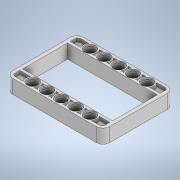
# Autodesk Inventor part: magazine-adapter
Saved by Autodesk Inventor 2021 (Build 250183000, 183)
## iProperties
Created: 2024-03-14
Part Number: magazine-adapter
Material: Generic
Document SubType Name: Modeling
Designer: 22hamfri
Density: 1 g/cm^3
Appearance: Default
Author: 22hamfri
Autodesk Inventor part; units mm, degrees
ref_plane "YZ Plane" through (0, 0, 0) normal (1, 0, 0) x (0, 1, 0)
ref_plane "XZ Plane" through (0, 0, 0) normal (0, 1, 0) x (-1, 0, 0)
ref_plane "XY Plane" through (0, 0, 0) normal (0, 0, 1) x (1, 0, 0)
sketch "Sketch1" plane through (0, 0, 0) normal (0, 1, 0) x (-1, 0, 0)
  line L0 (-25, 12.5) -> (25, 12.5)
  line L1 (25, 12.5) -> (25, -12.5)
  line L2 (25, -12.5) -> (-25, -12.5)
  line L3 (-25, -12.5) -> (-25, 12.5)
  line L4 (-25, 12.5) -> (25, -12.5) construction
  line L5 (25, 12.5) -> (-25, -12.5) construction
  line L6 (-27, 19.74) -> (27, 19.74)
  line L7 (27, 19.74) -> (27, -19.74)
  line L8 (27, -19.74) -> (-27, -19.74)
  line L9 (-27, -19.74) -> (-27, 19.74)
  line L10 (-27, 19.74) -> (27, -19.74) construction
  line L11 (27, 19.74) -> (-27, -19.74) construction
  circle A0 centre (0, -15.94) radius 2.575
  circle A1 centre (0, -15.94) radius 3.1
  circle A2 centre (0, -15.94) radius 3.8
  circle A3 centre (-7.97, -15.94) radius 2.575
  circle A4 centre (-7.97, -15.94) radius 3.1
  circle A5 centre (-7.97, -15.94) radius 3.8
  circle A6 centre (-15.94, -15.94) radius 2.575
  circle A7 centre (-15.94, -15.94) radius 3.1
  circle A8 centre (-15.94, -15.94) radius 3.8
  circle A9 centre (7.97, -15.94) radius 2.575
  circle A10 centre (7.97, -15.94) radius 3.1
  circle A11 centre (7.97, -15.94) radius 3.8
  circle A12 centre (0, -15.94) radius 2.575
  circle A13 centre (0, -15.94) radius 3.1
  circle A14 centre (0, -15.94) radius 3.8
  circle A15 centre (-7.97, -15.94) radius 2.575
  circle A16 centre (-7.97, -15.94) radius 3.1
  circle A17 centre (-7.97, -15.94) radius 3.8
  circle A18 centre (15.94, -15.94) radius 2.575
  circle A19 centre (15.94, -15.94) radius 3.1
  circle A20 centre (15.94, -15.94) radius 3.8
  circle A21 centre (7.97, -15.94) radius 2.575
  circle A22 centre (7.97, -15.94) radius 3.1
  circle A23 centre (7.97, -15.94) radius 3.8
  circle A24 centre (0, -15.94) radius 2.575
  circle A25 centre (0, -15.94) radius 3.1
  circle A26 centre (0, -15.94) radius 3.8
  line L12 (0, 0) -> (0, -19.74)
  line L13 (19.2075, -14) -> (25, -14)
  line L14 (25, -14) -> (25, -17.3718)
  line L15 (12.6725, -14) -> (11.2375, -14)
  line L16 (12.9151, -18.24) -> (10.9949, -18.24)
  line L17 (4.7025, -14) -> (3.2675, -14)
  line L18 (4.9451, -18.24) -> (3.0249, -18.24)
  line L19 (-3.2675, -14) -> (-4.7025, -14)
  line L20 (-3.0249, -18.24) -> (-4.9451, -18.24)
  line L21 (-11.2375, -14) -> (-12.6725, -14)
  line L22 (-10.9949, -18.24) -> (-12.9151, -18.24)
  line L23 (-19.2075, -14) -> (-25, -14)
  line L24 (-25, -14) -> (-25, -17.3718)
  arc A27 (23.2, -19.74) -> (27, -15.94) centre (23.2, -15.94) ccw
  arc A28 (23.2, -18.24) -> (25, -17.3718) centre (23.2, -15.94) ccw
  line L25 (23.2, -18.24) -> (18.9649, -18.24)
  arc A29 (-27, -15.94) -> (-23.2, -19.74) centre (-23.2, -15.94) ccw
  arc A30 (-25, -17.3718) -> (-23.2, -18.24) centre (-23.2, -15.94) ccw
  line L26 (-23.2, -18.24) -> (-18.9649, -18.24)
  line L27 (27, 0) -> (-27, 0)
  line L28 (25, 12.5) -> (-25, 12.5)
  line L29 (27, 19.74) -> (-27, 19.74)
  circle A31 centre (0, 15.94) radius 2.575
  circle A32 centre (0, 15.94) radius 3.1
  circle A33 centre (0, 15.94) radius 3.8
  circle A34 centre (-7.97, 15.94) radius 2.575
  circle A35 centre (-7.97, 15.94) radius 3.1
  circle A36 centre (-7.97, 15.94) radius 3.8
  circle A37 centre (-15.94, 15.94) radius 2.575
  circle A38 centre (-15.94, 15.94) radius 3.1
  circle A39 centre (-15.94, 15.94) radius 3.8
  circle A40 centre (7.97, 15.94) radius 2.575
  circle A41 centre (7.97, 15.94) radius 3.1
  circle A42 centre (7.97, 15.94) radius 3.8
  circle A43 centre (0, 15.94) radius 2.575
  circle A44 centre (0, 15.94) radius 3.1
  circle A45 centre (0, 15.94) radius 3.8
  circle A46 centre (-7.97, 15.94) radius 2.575
  circle A47 centre (-7.97, 15.94) radius 3.1
  circle A48 centre (-7.97, 15.94) radius 3.8
  circle A49 centre (15.94, 15.94) radius 2.575
  circle A50 centre (15.94, 15.94) radius 3.1
  circle A51 centre (15.94, 15.94) radius 3.8
  circle A52 centre (7.97, 15.94) radius 2.575
  circle A53 centre (7.97, 15.94) radius 3.1
  circle A54 centre (7.97, 15.94) radius 3.8
  circle A55 centre (0, 15.94) radius 2.575
  circle A56 centre (0, 15.94) radius 3.1
  circle A57 centre (0, 15.94) radius 3.8
  line L30 (19.2075, 14) -> (25, 14)
  line L31 (25, 14) -> (25, 17.3718)
  line L32 (12.6725, 14) -> (11.2375, 14)
  line L33 (12.9151, 18.24) -> (10.9949, 18.24)
  line L34 (4.7025, 14) -> (3.2675, 14)
  line L35 (4.9451, 18.24) -> (3.0249, 18.24)
  line L36 (-3.2675, 14) -> (-4.7025, 14)
  line L37 (-3.0249, 18.24) -> (-4.9451, 18.24)
  line L38 (-11.2375, 14) -> (-12.6725, 14)
  line L39 (-10.9949, 18.24) -> (-12.9151, 18.24)
  line L40 (-19.2075, 14) -> (-25, 14)
  line L41 (-25, 14) -> (-25, 17.3718)
  arc A58 (27, 15.94) -> (23.2, 19.74) centre (23.2, 15.94) ccw
  arc A59 (25, 17.3718) -> (23.2, 18.24) centre (23.2, 15.94) ccw
  line L42 (23.2, 18.24) -> (18.9649, 18.24)
  arc A60 (-23.2, 18.24) -> (-25, 17.3718) centre (-23.2, 15.94) ccw
  arc A61 (-23.2, 19.74) -> (-27, 15.94) centre (-23.2, 15.94) ccw
  line L43 (-23.2, 18.24) -> (-18.9649, 18.24)
  point P0 (0, 0)
  point P1 (0, 19.74)
  point P2 (-23.2, 19.74)
  point P3 (-27, 15.94)
  point P4 (-27, -15.94)
  point P5 (-23.2, -19.74)
  point P6 (-3.2675, -14)
  point P7 (-3.0249, -18.24)
  point P8 (4.9451, -18.24)
  point P9 (3.0249, -18.24)
  point P10 (3.2675, -14)
  point P11 (4.7025, -14)
  point P12 (10.9949, -18.24)
  point P13 (11.2375, -14)
  dimension "d0" = 25
  dimension "d1" = 50
  dimension "d2" = 2
  dimension "d3" = 5.15
  dimension "d4" = 6.2
  dimension "d5" = 0.7
  dimension "d8" = 7.97
  dimension "d11" = 7.97
  dimension "d14" = 2
  dimension "d15" = 1.5
  dimension "d17" = 3.8
  dimension "d18" = 1.5
  dimension "d19" = 1.5
  dimension "d26" = 31.88
  constraints: 88 end point, 62 centre point, 56 point on circle, 47 symmetric about line, 12 collinear, 11 parallel, 10 point on line, 9 midpoint, 6 horizontal, 5 perpendicular, 3 tangent, 65 other
  measures "d0" distance between parallel lines of L2 L0
  measures "d1" distance between parallel lines of L1 L3
  measures "d2" distance between parallel lines of L7 L1
  measures "d3" diameter of A0
  measures "d4" diameter of A1
  measures "d5" radial gap between concentric circles of A1 A2
  measures "d8" distance of A0.centre A3.centre
  measures "d11" distance of A0.centre A9.centre
  measures "d14" distance between parallel lines of L3 L9
  measures "d15" distance between parallel lines of L13 L2
  measures "d17" radius of A27
  measures "d18" radial gap between concentric circles of A27 A28
  measures "d19" distance between parallel lines of L8 L25
  measures "d26" distance of A56.centre A0.centre
extrude "Extrusion1" add sketch "Sketch1" against normal mid plane 7.76 contours L3 L27 L9 A61 L6 A39 L43 A60 L41 L40 L0 | A39 L0 | L3 L2 A8 L23 L24 A30 L26 L8 A29 L9 L27 | A39 L38 A36 L0 | A36 L0 | L2 A8 | L27 L7 A27 L8 A20 L25 A28 L14 L13 L2 L1 | L1 L0 A51 L30 L31 A59 L42 L6 A58 L7 L27 | A36 L36 A33 L0 | L6 A36 L39 A39 | L2 A5 L21 A8 | A2 L12 A1 L2 | L2 A11 L17 A2 | A2 L19 A5 L2 | L2 L12 A1 A2 | A33 L0 | L6 A33 L37 A36 | L2 A5 | L2 A11 | L0 A51 | A20 L2 | A8 L22 A5 L8 | A33 L34 A42 L0 | L6 A42 L35 A33 | L2 A20 L15 A11 | A2 L8 A5 L20 | L0 A42 L32 A51 | A42 L0 | L6 A51 L33 A42 | A11 L8 A2 L18 | L8 A11 L16 A20 picked at (-15.8154, 12.6209) picked at (-7.8454, 12.6209) picked at (-16.0646, -12.6209) picked at (0.1246, 12.6209) picked at (-7.8454, -12.6209) picked at (7.8454, -12.6209) picked at (16.0646, 12.6209) picked at (15.8154, -12.6209) picked at (8.0946, 12.6209)
extrude "Extrusion2" add sketch "Sketch1" against normal mid plane 6.16 contours L12 A0 A1 | A1 L12 A0 | A4 | A7 | A10 | A19 | A32 | A35 | A38 | A41 | A50
extrude "Extrusion3" add sketch "Sketch1" along normal mid plane 4 contours L40 L41 A60 L43 A39 | A39 L39 A36 L38 | A8 L26 A30 L24 L23 | A36 L37 A33 L36 | L21 A5 L22 A8 | L17 A11 L18 A2 | A2 L20 A5 L19 | A51 L42 A59 L31 L30 | L13 L14 A28 L25 A20 | A33 L35 A42 L34 | L15 A20 L16 A11 | L32 A42 L33 A51
equation "\"d14\" = d2"
equation "\"d18\" = d15"
equation "\"d19\" = d15"
equation "\"d16\" = d15"
body "Solid1"
